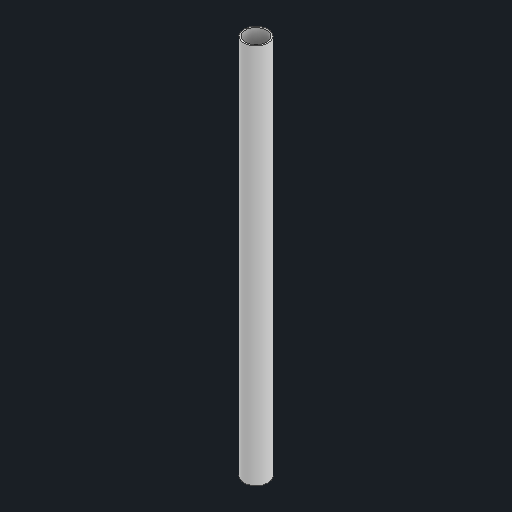
# Autodesk Inventor part: cradle_post
Saved by Autodesk Inventor 2025 (Build 290162010, 162A)
## iProperties
Created: 2024-06-21
Part Number: cradle_post
Material: Generic
Document SubType Name: Modeling
Designer: mihir
Density: 1 g/cm^3
Appearance: Default
Author: mihir
Autodesk Inventor part; units mm, degrees
ref_plane "YZ Plane" through (0, 0, 0) normal (1, 0, 0) x (0, 1, 0)
ref_plane "XZ Plane" through (0, 0, 0) normal (0, 1, 0) x (-1, 0, 0)
ref_plane "XY Plane" through (0, 0, 0) normal (0, 0, 1) x (1, 0, 0)
sketch "Sketch1" plane through (0, 0, 0) normal (0, 1, 0) x (-1, 0, 0)
  circle A0 centre (0, 0) radius 3.25
  circle A1 centre (0, 0) radius 5.1
  dimension "d0" = 10.2
  dimension "d1" = 6.5
  constraints: 2 centre point, 2 coincident
  measures "d0" diameter of A1
  measures "d1" diameter of A0
extrude "Extrusion1" add sketch "Sketch1" along normal blind 160
sketch "Sketch2" plane through (0, 160, 0) normal (0, 1, 0) x (1, 0, 0)
  circle A0 centre (0, 0) radius 5.1 projected
  circle A1 centre (0, 0) radius 4.45
  dimension "d4" = 0.65
  constraints: 1 centre point, 1 coincident
  measures "d4" radial gap between concentric circles of A0 A1
extrude "Extrusion2" cut sketch "Sketch2" against normal blind 10 contours A1
equation "\"d0\" = post_diameter"
equation "\"d1\" = rod_diameter + rod_free_tolerance"
equation "\"d2\" = post_height"
equation "\"d4\" = post_wall_diameter"
equation "\"d5\" = cradle_holder_peg_depth"
equation "\"post_diameter\" = 10.2"
equation "\"rod_diameter\" = 6"
equation "\"rod_free_tolerance\" = 0.5"
equation "\"post_height\" = 160"
equation "\"cradle_holder_peg_depth\" = 10"
equation "\"post_wall_diameter\" = 0.65"
body "Solid1"
